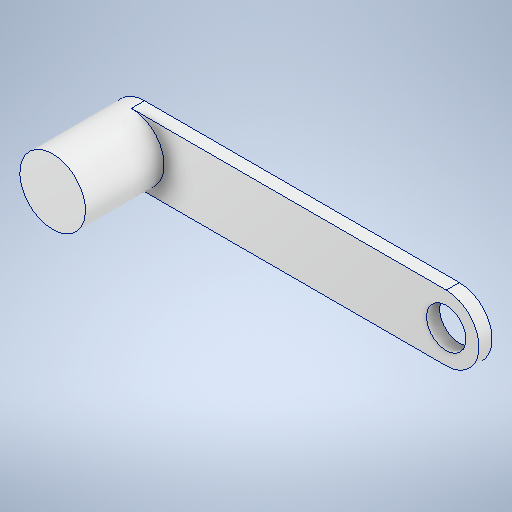
# Autodesk Inventor part: L1
Saved by Autodesk Inventor 2025 (Build 290162000, 162)
## iProperties
Created: 2023-05-06
Part Number: L1
Material: Aluminio 6061
Document SubType Name: Modeling
Designer: Miguel Ángel
Density: 2.7 g/cm^3
Appearance: Aluminio - Plano
Author: Miguel Ángel
Autodesk Inventor part; units mm, degrees
ref_plane "YZ Plane" through (0, 0, 0) normal (1, 0, 0) x (0, 1, 0)
ref_plane "XZ Plane" through (0, 0, 0) normal (0, 1, 0) x (-1, 0, 0)
ref_plane "XY Plane" through (0, 0, 0) normal (0, 0, 1) x (1, 0, 0)
sketch "Boceto1" plane through (0, 0, 0) normal (0, 0, 1) x (1, 0, 0)
  line L0 (-4.4214, -2.4997) -> (115.5786, -2.4997) construction
  line L1 (-4.4214, -14.9997) -> (115.5786, -14.9997)
  line L2 (115.5786, 10.0003) -> (-4.4214, 10.0003)
  arc A0 (-4.4214, 10.0003) -> (-4.4214, -14.9997) centre (-4.4214, -2.4997) ccw
  arc A1 (115.5786, -14.9997) -> (115.5786, 10.0003) centre (115.5786, -2.4997) ccw
  circle A2 centre (115.5786, -2.4997) radius 7.5
  point P0 (0, 0)
  point P1 (55.5786, -2.4997)
  dimension "d3" = 120
  dimension "d4" = 25
  dimension "d5" = 15
  constraints: 8 end point, 4 point on circle, 4 tangent, 3 centre point, 1 coincident, 1 horizontal, 1 midpoint, 1 parallel
  measures "d3" distance of L0.start L0.end
  measures "d4" diameter of A1
  measures "d5" diameter of A2
extrude "Extrusión1" add sketch "Boceto1" along normal blind 5
sketch "Boceto4" plane through (0, 0, 5) normal (0, 0, 1) x (1, 0, 0)
  arc A0 (-4.4214, 10.0003) -> (-4.4214, -14.9997) centre (-4.4214, -2.4997) ccw projected
  circle A1 centre (-4.4214, -2.4997) radius 12.5
  point P0 (0, 0)
  point P1 (-4.4214, -14.9997)
  dimension "d12" = 25
  constraints: 1 centre point, 1 coincident
  measures "d12" diameter of A1
extrude "Extrusión3" add sketch "Boceto4" along normal blind 30
